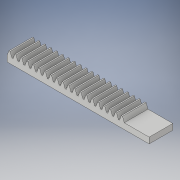
# Autodesk Inventor part: rack
Saved by Autodesk Inventor 2019 (Build 230136000, 136)
## iProperties
Created: 2021-01-03
Part Number: rack
Material: Типовые
Document SubType Name: Modeling
Designer: Professional
Density: 1 g/cm^3
Appearance: По умолчанию
Author: Professional
Autodesk Inventor part; units mm, degrees
ref_plane "YZ Plane" through (0, 0, 0) normal (1, 0, 0) x (0, 1, 0)
ref_plane "XZ Plane" through (0, 0, 0) normal (0, 1, 0) x (-1, 0, 0)
ref_plane "XY Plane" through (0, 0, 0) normal (0, 0, 1) x (1, 0, 0)
sketch "Эскиз1" plane through (0, 0, 0) normal (0, 0, 1) x (1, 0, 0)
  line L0 (-60, 0) -> (60, 0)
  line L1 (60, 0) -> (60, 5)
  line L2 (60, 5) -> (-60, 5)
  line L3 (-60, 5) -> (-60, 0)
  point P0 (0, 0)
  point P1 (0, 0)
  dimension "d0" = 5
  dimension "d1" = 120
  constraints: 8 end point, 2 parallel, 1 coincident, 1 horizontal, 1 midpoint, 1 perpendicular
  measures "d0" distance between parallel lines of L0 L2
  measures "d1" distance between parallel lines of L1 L3
extrude "Выдавливание1" add sketch "Эскиз1" along normal mid plane 20
sketch "Эскиз3" plane through (0, 0, 0) normal (0, 0, 1) x (1, 0, 0)
  line L0 (-60, 5) -> (-58.5441, 9)
  line L1 (-58.5441, 9) -> (-57.5, 9)
  line L2 (-57.5, 9) -> (-56.0441, 5)
  line L3 (-60, 5) -> (60, 5) projected
  line L4 (-59.2721, 7) -> (-56.7721, 7) construction
  point P0 (0, 0)
  dimension "d4" = 40
  dimension "d5" = 4
  dimension "d6" = 2.5
  constraints: 8 end point, 2 midpoint, 1 equal length, 1 horizontal, 1 point on line
  measures "d4" angle of L0 L2
  measures "d5" distance between parallel lines of L3 L1
  measures "d6" distance of L4.start L4.end
extrude "Выдавливание2" add sketch "Эскиз3" against normal up to surface (20 mm away) from surface at 10
pattern_linear "Прямоуг.массив1" count 20 spacing 5 along (1, 0, 0) of "Выдавливание2"
